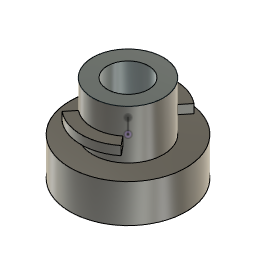
F16 Adapter v2 (Autodesk Fusion 360 design; units mm, degrees)
Autodesk Fusion 360 part; units mm, degrees
sketch "Sketch1" plane through (0, 0, 0) normal (0, 0, 1) x (1, 0, 0)
  circle A0 centre (0, 0) radius 12
  dimension "d1" = 24
  constraint coincident A0.centre origin
  measures "d1" diameter of A0
extrude "Extrude1" add sketch "Sketch1" along normal blind 16.75 makes body 1
sketch "Sketch2" plane through (0, 0, 0) normal (0, 0, 1) x (1, 0, 0)
  circle A0 centre (0, 0) radius 19.75
  dimension "d4" = 39.5
  constraint coincident A0.centre origin
  measures "d4" diameter of A0
extrude "Extrude2" add sketch "Sketch2" against normal blind 13 bodies 1
sketch "Sketch3" plane through (0, 0, 0) normal (0, 1, 0) x (1, 0, 0)
  line L0 (0, 0) -> (0, -4.94)
  dimension "d7" = 4.94
  constraint coincident L0.start origin
  constraint vertical L0
  measures "d7" distance of L0.start L0.end
sketch "Sketch4" plane through (0, 0, 16.75) normal (0, 0, 1) x (-1, 0, 0)
  circle A0 centre (0, 0) radius 12
sketch "Sketch5" plane through (0, 0, 0) normal (0, 1, 0) x (1, 0, 0)
sketch "Sketch6" plane through (0, 0, 0) normal (0, 0, 1) x (1, 0, 0)
  circle A0 centre (0, 0) radius 16
  dimension "d9" = 32
  constraint coincident A0.centre origin
  measures "d9" diameter of A0
extrude "Extrude3" add sketch "Sketch6" along normal blind 3 separate body makes body 2
move_body "Move1" bodies 2 to x (1, 0, 0) y (0, 1, 0) z (0, 0, 1) at (0, 0, 4.94)
sketch "Sketch7" plane through (0, 0, 7.94) normal (0, 0, 1) x (-1, 0, 0)
  circle A0 centre (0, 0) radius 16
  line L0 (0, 0) -> (13, 16)
  line L1 (0, -2.5) -> (0, -20)
  line L2 (0, 0) -> (-13, 16)
  line L3 (-20, 0) -> (-2.5, 0)
  line L4 (0, 0) -> (13, -16)
  line L5 (0, 0) -> (-13, -16)
  line L6 (-13, 16) -> (-22, 6)
  line L7 (-22, 6) -> (-13, -16)
  line L8 (13, 16) -> (27, 0)
  line L9 (27, 0) -> (13, -16)
  constraint coincident A0.centre L0.start
  constraint symmetric A0.centre L1 L0.start
  constraint symmetric L0.end L1 L2.end
  constraint symmetric A0.centre L3 L0.start
  constraint symmetric L0.end L3 L4.end
  constraint symmetric L2.end L3 L5.end
extrude "Extrude4" cut sketch "Sketch7" against normal blind 4 contours A0 L0 L4 | A0 L0 L4 L8 L9 | A0 L2 L5 | A0 L2 L3 L6 L7 | A0 L3 L5 L7 bodies 2
sketch "Sketch8" plane through (0, 0, 16.75) normal (0, 0, 1) x (-1, 0, 0)
  circle A0 centre (0, 0) radius 7
  dimension "d14" = 14
  constraint coincident A0.centre origin
  measures "d14" diameter of A0
extrude "Extrude5" cut sketch "Sketch8" against normal blind 33 bodies 1 2 makes body 3 at (-4.4893, -12.169, 7.94)
combine "Combine1" operation add target body 1 tool bodies 2 3
